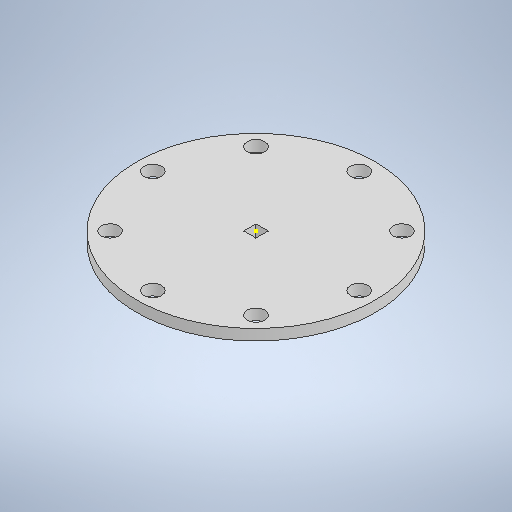
# Autodesk Inventor part: SCARA swivel base
Saved by Autodesk Inventor 2025.2 (Build 292293000, 293)
## iProperties
Created: 2025-01-25
Part Number: SCARA swivel base
Material: Generic
Document SubType Name: Modeling
Designer: caomi
Density: 1 g/cm^3
Appearance: Default
Author: caomi
Autodesk Inventor part; units mm, degrees
ref_plane "YZ Plane" through (0, 0, 0) normal (1, 0, 0) x (0, 1, 0)
ref_plane "XZ Plane" through (0, 0, 0) normal (0, 1, 0) x (-1, 0, 0)
ref_plane "XY Plane" through (0, 0, 0) normal (0, 0, 1) x (1, 0, 0)
sketch "Sketch1" plane through (0, 0, 0) normal (1, 0, 0) x (0, 1, 0)
  line L0 (0, 0) -> (0, -17.5)
  line L1 (15, -55) -> (20, -55)
  line L2 (20, -55) -> (20, 0)
  line L3 (20, 0) -> (0, 0)
  line L4 (0, -17.5) -> (15, -17.5)
  line L5 (15, -17.5) -> (15, -55)
  dimension "d2" = 17.5
  dimension "d3" = 55
  dimension "d4" = 20
  dimension "d11" = 15
  constraints: 12 end point, 3 vertical, 2 horizontal, 1 perpendicular
  measures "d2" distance of L0.end L0.start
  measures "d3" vertical distance of L1.start L0.start
  measures "d4" distance of L2.end L0.start
  measures "d11" distance of L0.end L4.end
revolve "Revolution1" add sketch "Sketch1" angle 360 about axis through (0, 20, 0) along (0, -1, 0)
sketch "Sketch2" plane through (0, 20, 0) normal (0, 1, 0) x (1, 0, 0)
  line L0 (2.8, -2.8) -> (-2.8, -2.8)
  line L1 (-2.8, -2.8) -> (-2.8, 2.8)
  line L2 (-2.8, 2.8) -> (2.8, 2.8)
  line L3 (2.8, 2.8) -> (2.8, -2.8)
  line L4 (2.8, -2.8) -> (-2.8, 2.8) construction
  line L5 (-2.8, -2.8) -> (2.8, 2.8) construction
  point P0 (0, 0)
  point P1 (0, 0)
  dimension "d7" = 5.6
  constraints: 12 end point, 2 parallel, 2 perpendicular, 1 coincident, 1 horizontal, 1 midpoint
  measures "d7" distance of L0.end L1.end
extrude "Extrusion1" cut sketch "Sketch2" against normal up to surface (20 mm away)
sketch "Sketch3" plane through (0, 0, 0) normal (1, 0, 0) x (0, 1, 0)
  point P0 (0, 0)
sketch "Sketch4" plane through (0, 0, 0) normal (1, 0, 0) x (0, 1, 0)
  line L0 (11.0047, 34.4347) -> (4.1371, 14.8288)
  line L1 (11.0047, 34.4347) -> (15.5479, 34.4347)
  point P0 (0, 0)
  constraints: 4 end point, 1 horizontal
extrude "Rib1" add sketch "Sketch4" along normal mid plane 3 rib yes fills toward (13.2763, 34.3847) open curves L1 L0
pattern_circular "Circular Pattern1" count 6 over 360 about axis through (0, 7.5, 0) along (0, -1, 0) of "Rib1"
sketch "Sketch5" plane through (0, 0, 0) normal (0, -1, 0) x (1, 0, 0)
  line L0 (17.4356, 1.5) -> (27.4356, 1.5)
  circle A0 centre (0, 0) radius 17.5 projected
  line L1 (17.4356, -1.5) -> (27.4356, -1.5)
  line L2 (-3.235, 0) -> (43.5251, 0) construction
  circle A1 centre (27.4356, 0) radius 1.5
  circle A2 centre (0, 0) radius 17.5
  point P0 (0, 0)
  point P1 (22.4356, -1.5)
  dimension "d21" = 3
  dimension "d22" = 10
  constraints: 6 end point, 4 point on circle, 3 horizontal, 2 centre point, 2 point on line, 1 coincident, 1 midpoint, 1 tangent, 1 other
  measures "d21" distance from line of point (22.436, -1.5) L0
  measures "d22" distance of L1.start L1.end
extrude "Extrusion2" add sketch "Sketch5" against normal up to surface (15 mm away) contours L0 A1 L1 A0 | A1
sketch "Sketch6" plane through (0, 20, 0) normal (0, 1, 0) x (1, 0, 0)
  point P0 (0, 0)
extrude "Extrusion3" cut sketch "Sketch5" against normal blind 2 contours L0 A1 L1 A0 | A1
sketch "Sketch7" plane through (0, 15, 0) normal (0, -1, 0) x (1, 0, 0)
  circle A0 centre (47.5, 0) radius 4.0602
  point P0 (0, 0)
  dimension "d27" = 47.5
  constraints: 1 centre point, 1 horizontal alignment
  measures "d27" distance of A0.centre point (0, 0)
extrude "Extrusion4" cut sketch "Sketch7" against normal blind 47.5
pattern_circular "Circular Pattern2" count 8 over 360 about axis through (0, 17.5, 0) along (0, -1, 0) of "Extrusion4"
equation "\"d28\" = d27"
body "Solid1"
